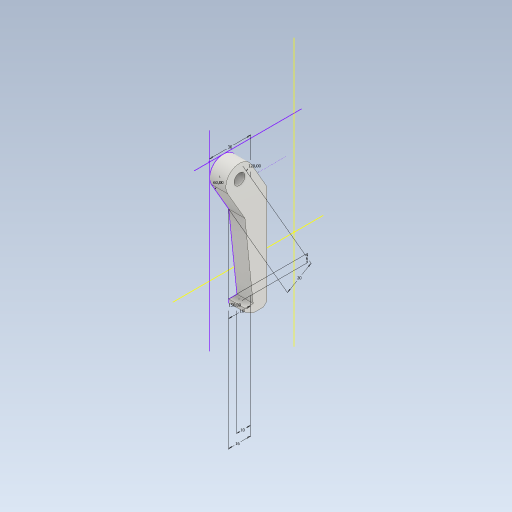
# Autodesk Inventor part: Abzieher_Klaue1
Saved by Autodesk Inventor 2024.3 (Build 283343000, 343)
## iProperties
Created: 2025-08-29
Part Number: Abzieher_Klaue1
Material: 1.0038 S235JR
Document SubType Name: Modeling
Designer: Dickert.Jonas
Density: 7.86 g/cm^3
Appearance: Stahl
Author: Dickert.Jonas
Autodesk Inventor part; units mm, degrees
ref_plane "YZ Plane" through (0, 0, 0) normal (1, 0, 0) x (0, 1, 0)
ref_plane "XZ Plane" through (0, 0, 0) normal (0, 1, 0) x (-1, 0, 0)
ref_plane "XY Plane" through (0, 0, 0) normal (0, 0, 1) x (1, 0, 0)
sketch "Skizze1" plane through (0, 0, 0) normal (1, 0, 0) x (0, 1, 0)
  line L0 (-88.8183, 0) -> (21.3265, 0) projected
  line L1 (0, -72.4192) -> (0, 123.5808) projected
  line L2 (-61.844, -44.4192) -> (-61.844, 95.5808)
  line L3 (-31.844, 50.9398) -> (-31.844, -24.4192)
  line L4 (-41.844, -18.4192) -> (-47.844, -18.4192)
  line L5 (-41.844, -24.4192) -> (-47.844, -20.9551)
  line L6 (-41.844, -24.4192) -> (-34.9129, -24.4192) construction
  line L7 (-31.844, 50.9398) -> (-43.1838, 70.5808)
  line L8 (-31.844, 50.9398) -> (-5.6477, 50.9398) construction
  circle A0 centre (-51.844, 65.5808) radius 10
  line L9 (-60.5043, 60.5808) -> (-47.844, 38.6526)
  line L10 (-61.844, 62.7769) -> (-45.1591, 62.7769) construction
  line L11 (-47.844, 38.6526) -> (-41.844, -18.4192)
  line L12 (-31.844, -24.4192) -> (-41.844, -24.4192)
  line L13 (-47.844, -20.9551) -> (-47.844, -18.4192)
  line L14 (-73.0833, 75.5808) -> (5.5916, 75.5808)
  point P0 (0, 0)
  point P1 (-61.844, 75.5808)
  point P2 (-37.5139, 60.7603)
  dimension "d0" = 150
  dimension "d1" = 120
  dimension "d2" = 60
  dimension "d3" = 6
  dimension "d4" = 16
  dimension "d5" = 10
  dimension "d6" = 20
  dimension "d7" = 30
  dimension "d8" = 16
  constraints: 26 end point, 4 horizontal, 2 point on circle, 2 tangent, 1 centre point, 1 coincident, 1 midpoint
  measures "d0" angle of L6 L5
  measures "d1" angle of L8 L7
  measures "d2" angle of L9 L10
  measures "d3" distance of L12.end L11.end
  measures "d4" horizontal distance of L13.start L3.end
  measures "d5" distance of L12.end L3.end
  measures "d6" distance from line of L9 point (-37.514, 60.76)
  measures "d7" distance between parallel lines of L2 L3
  measures "d8" distance from line of L3 L11.start
extrude "Extrusion1" add sketch "Skizze1" along normal blind 12 contours L11 L9 A0 L7 L3 L0 | L0 L3 L12 L5 L13 L4 L11 | A0
hole "Bohrung1" at (0, -51.844, 65.5808) direction (1, 0, 0) diameter 8 end through all
chamfer "Fasen1" distance 2.5 angle 45 1 edges at (6, -31.844, -24.4192) measured on face at (4, -38.5107, -24.4192)
